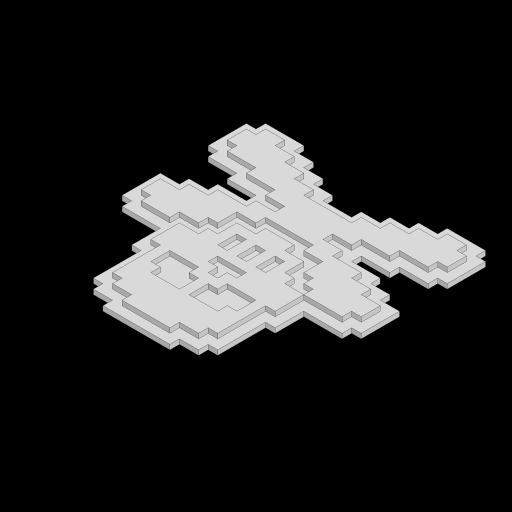
# Autodesk Inventor part: PKSkull
Saved by Autodesk Inventor 2023 (Build 270158000, 158)
## iProperties
Created: 2023-09-16
Part Number: PKSkull
Material: Generic
Document SubType Name: Modeling
Designer: tandu
Density: 1 g/cm^3
Appearance: Default
Author: tandu
Autodesk Inventor part; units mm, degrees
ref_plane "YZ Plane" through (0, 0, 0) normal (1, 0, 0) x (0, 1, 0)
ref_plane "XZ Plane" through (0, 0, 0) normal (0, 1, 0) x (-1, 0, 0)
ref_plane "XY Plane" through (0, 0, 0) normal (0, 0, 1) x (1, 0, 0)
sketch "Sketch1" plane through (0, 0, 0) normal (0, 1, 0) x (-1, 0, 0)
  line L0 (3708.4, 6832.6) -> (3708.4, 6705.6)
  line L1 (3708.4, 6705.6) -> (3454.4, 6705.6)
  line L2 (3454.4, 6705.6) -> (3200.4, 6705.6)
  line L3 (3200.4, 6705.6) -> (3200.4, 6578.6)
  line L4 (3200.4, 6578.6) -> (3200.4, 6451.6)
  line L5 (3200.4, 6451.6) -> (3073.4, 6451.6)
  line L6 (3073.4, 6451.6) -> (2946.4, 6451.6)
  line L7 (2946.4, 6451.6) -> (2946.4, 5816.6)
  line L8 (2946.4, 5816.6) -> (2946.4, 5181.6)
  line L9 (2946.4, 5181.6) -> (2819.4, 5181.6)
  line L10 (2819.4, 5181.6) -> (2692.4, 5181.6)
  line L11 (2692.4, 5181.6) -> (2692.4, 4800.6)
  line L12 (2692.4, 4800.6) -> (2692.4, 4419.6)
  line L13 (2692.4, 4419.6) -> (2184.4, 4419.6)
  line L14 (2184.4, 4419.6) -> (1676.4, 4419.6)
  line L15 (1676.4, 4419.6) -> (1676.4, 4292.6)
  line L16 (1676.4, 4292.6) -> (1676.4, 4165.6)
  line L17 (1676.4, 4165.6) -> (1549.4, 4165.6)
  line L18 (1549.4, 4165.6) -> (1422.4, 4165.6)
  line L19 (1422.4, 4165.6) -> (1422.4, 3657.6)
  line L20 (1422.4, 3657.6) -> (1422.4, 3149.6)
  line L21 (1422.4, 3149.6) -> (1676.4, 3149.6)
  line L22 (1676.4, 3149.6) -> (1930.4, 3149.6)
  line L23 (1930.4, 3149.6) -> (1930.4, 3022.6)
  line L24 (1930.4, 3022.6) -> (1930.4, 2895.6)
  line L25 (1930.4, 2895.6) -> (2184.4, 2895.6)
  line L26 (2184.4, 2895.6) -> (2438.4, 2895.6)
  line L27 (2438.4, 2895.6) -> (2438.4, 2768.6)
  line L28 (2438.4, 2768.6) -> (2438.4, 2641.6)
  line L29 (2438.4, 2641.6) -> (2819.4, 2641.6)
  line L30 (2819.4, 2641.6) -> (3200.4, 2641.6)
  line L31 (3200.4, 2641.6) -> (3200.4, 2514.6)
  line L32 (3200.4, 2514.6) -> (3200.4, 2387.6)
  line L33 (3200.4, 2387.6) -> (2819.4, 2387.6)
  line L34 (2819.4, 2387.6) -> (2438.4, 2387.6)
  line L35 (2438.4, 2387.6) -> (2438.4, 2260.6)
  line L36 (2438.4, 2260.6) -> (2438.4, 2133.6)
  line L37 (2438.4, 2133.6) -> (2057.4, 2133.6)
  line L38 (2057.4, 2133.6) -> (1676.4, 2133.6)
  line L39 (1676.4, 2133.6) -> (1676.4, 2006.6)
  line L40 (1676.4, 2006.6) -> (1676.4, 1879.6)
  line L41 (1676.4, 1879.6) -> (1549.4, 1879.6)
  line L42 (1549.4, 1879.6) -> (1422.4, 1879.6)
  line L43 (1422.4, 1879.6) -> (1422.4, 1371.6)
  line L44 (1422.4, 1371.6) -> (1422.4, 863.6)
  line L45 (1422.4, 863.6) -> (1549.4, 863.6)
  line L46 (1549.4, 863.6) -> (1676.4, 863.6)
  line L47 (1676.4, 863.6) -> (1676.4, 736.6)
  line L48 (1676.4, 736.6) -> (1676.4, 609.6)
  line L49 (1676.4, 609.6) -> (2184.4, 609.6)
  line L50 (2184.4, 609.6) -> (2692.4, 609.6)
  line L51 (2692.4, 609.6) -> (2692.4, 736.6)
  line L52 (2692.4, 736.6) -> (2692.4, 863.6)
  line L53 (2692.4, 863.6) -> (2946.4, 863.6)
  line L54 (2946.4, 863.6) -> (3200.4, 863.6)
  line L55 (3200.4, 863.6) -> (3200.4, 990.6)
  line L56 (3200.4, 990.6) -> (3200.4, 1117.6)
  line L57 (3200.4, 1117.6) -> (3454.4, 1117.6)
  line L58 (3454.4, 1117.6) -> (3708.4, 1117.6)
  line L59 (3708.4, 1117.6) -> (3708.4, 1244.6)
  line L60 (3708.4, 1244.6) -> (3708.4, 1371.6)
  line L61 (3708.4, 1371.6) -> (3962.4, 1371.6)
  line L62 (3962.4, 1371.6) -> (4216.4, 1371.6)
  line L63 (4216.4, 1371.6) -> (4216.4, 1498.6)
  line L64 (4216.4, 1498.6) -> (4216.4, 1625.6)
  line L65 (4216.4, 1625.6) -> (4597.4, 1625.6)
  line L66 (4597.4, 1625.6) -> (4978.4, 1625.6)
  line L67 (4978.4, 1625.6) -> (4978.4, 1498.6)
  line L68 (4978.4, 1498.6) -> (4978.4, 1371.6)
  line L69 (4978.4, 1371.6) -> (5232.4, 1371.6)
  line L70 (5232.4, 1371.6) -> (5486.4, 1371.6)
  line L71 (5486.4, 1371.6) -> (5486.4, 1244.6)
  line L72 (5486.4, 1244.6) -> (5486.4, 1117.6)
  line L73 (5486.4, 1117.6) -> (5740.4, 1117.6)
  line L74 (5740.4, 1117.6) -> (5994.4, 1117.6)
  line L75 (5994.4, 1117.6) -> (5994.4, 990.6)
  line L76 (5994.4, 990.6) -> (5994.4, 863.6)
  line L77 (5994.4, 863.6) -> (6248.4, 863.6)
  line L78 (6248.4, 863.6) -> (6502.4, 863.6)
  line L79 (6502.4, 863.6) -> (6502.4, 736.6)
  line L80 (6502.4, 736.6) -> (6502.4, 609.6)
  line L81 (6502.4, 609.6) -> (7010.4, 609.6)
  line L82 (7010.4, 609.6) -> (7518.4, 609.6)
  line L83 (7518.4, 609.6) -> (7518.4, 736.6)
  line L84 (7518.4, 736.6) -> (7518.4, 863.6)
  line L85 (7518.4, 863.6) -> (7645.4, 863.6)
  line L86 (7645.4, 863.6) -> (7772.4, 863.6)
  line L87 (7772.4, 863.6) -> (7772.4, 1371.6)
  line L88 (7772.4, 1371.6) -> (7772.4, 1879.6)
  line L89 (7772.4, 1879.6) -> (7645.4, 1879.6)
  line L90 (7645.4, 1879.6) -> (7518.4, 1879.6)
  line L91 (7518.4, 1879.6) -> (7518.4, 2006.6)
  line L92 (7518.4, 2006.6) -> (7518.4, 2133.6)
  line L93 (7518.4, 2133.6) -> (7137.4, 2133.6)
  line L94 (7137.4, 2133.6) -> (6756.4, 2133.6)
  line L95 (6756.4, 2133.6) -> (6756.4, 2260.6)
  line L96 (6756.4, 2260.6) -> (6756.4, 2387.6)
  line L97 (6756.4, 2387.6) -> (6375.4, 2387.6)
  line L98 (6375.4, 2387.6) -> (5994.4, 2387.6)
  line L99 (5994.4, 2387.6) -> (5994.4, 2514.6)
  line L100 (5994.4, 2514.6) -> (5994.4, 2641.6)
  line L101 (5994.4, 2641.6) -> (6375.4, 2641.6)
  line L102 (6375.4, 2641.6) -> (6756.4, 2641.6)
  line L103 (6756.4, 2641.6) -> (6756.4, 2768.6)
  line L104 (6756.4, 2768.6) -> (6756.4, 2895.6)
  line L105 (6756.4, 2895.6) -> (7010.4, 2895.6)
  line L106 (7010.4, 2895.6) -> (7264.4, 2895.6)
  line L107 (7264.4, 2895.6) -> (7264.4, 3022.6)
  line L108 (7264.4, 3022.6) -> (7264.4, 3149.6)
  line L109 (7264.4, 3149.6) -> (7518.4, 3149.6)
  line L110 (7518.4, 3149.6) -> (7772.4, 3149.6)
  line L111 (7772.4, 3149.6) -> (7772.4, 3657.6)
  line L112 (7772.4, 3657.6) -> (7772.4, 4165.6)
  line L113 (7772.4, 4165.6) -> (7645.4, 4165.6)
  line L114 (7645.4, 4165.6) -> (7518.4, 4165.6)
  line L115 (7518.4, 4165.6) -> (7518.4, 4292.6)
  line L116 (7518.4, 4292.6) -> (7518.4, 4419.6)
  line L117 (7518.4, 4419.6) -> (7010.4, 4419.6)
  line L118 (7010.4, 4419.6) -> (6502.4, 4419.6)
  line L119 (6502.4, 4419.6) -> (6502.4, 4800.6)
  line L120 (6502.4, 4800.6) -> (6502.4, 5181.6)
  line L121 (6502.4, 5181.6) -> (6375.4, 5181.6)
  line L122 (6375.4, 5181.6) -> (6248.4, 5181.6)
  line L123 (6248.4, 5181.6) -> (6248.4, 5816.6)
  line L124 (6248.4, 5816.6) -> (6248.4, 6451.6)
  line L125 (6248.4, 6451.6) -> (6121.4, 6451.6)
  line L126 (6121.4, 6451.6) -> (5994.4, 6451.6)
  line L127 (5994.4, 6451.6) -> (5994.4, 6578.6)
  line L128 (5994.4, 6578.6) -> (5994.4, 6705.6)
  line L129 (5994.4, 6705.6) -> (5740.4, 6705.6)
  line L130 (5740.4, 6705.6) -> (5486.4, 6705.6)
  line L131 (5486.4, 6705.6) -> (5486.4, 6832.6)
  line L132 (5486.4, 6832.6) -> (5486.4, 6959.6)
  line L133 (5486.4, 6959.6) -> (4597.4, 6959.6)
  line L134 (4597.4, 6959.6) -> (3708.4, 6959.6)
  line L135 (3708.4, 6959.6) -> (3708.4, 6832.6)
  line L136 (5232.4, 6578.6) -> (5232.4, 6451.6)
  line L137 (5232.4, 6451.6) -> (5486.4, 6451.6)
  line L138 (5486.4, 6451.6) -> (5740.4, 6451.6)
  line L139 (5740.4, 6451.6) -> (5740.4, 6324.6)
  line L140 (5740.4, 6324.6) -> (5740.4, 6197.6)
  line L141 (5740.4, 6197.6) -> (5867.4, 6197.6)
  line L142 (5867.4, 6197.6) -> (5994.4, 6197.6)
  line L143 (5994.4, 6197.6) -> (5994.4, 5562.6)
  line L144 (5994.4, 5562.6) -> (5994.4, 4927.6)
  line L145 (5994.4, 4927.6) -> (6121.4, 4927.6)
  line L146 (6121.4, 4927.6) -> (6248.4, 4927.6)
  line L147 (6248.4, 4927.6) -> (6248.4, 4546.6)
  line L148 (6248.4, 4546.6) -> (6248.4, 4165.6)
  line L149 (6248.4, 4165.6) -> (5994.4, 4165.6)
  line L150 (5994.4, 4165.6) -> (5740.4, 4165.6)
  line L151 (5740.4, 4165.6) -> (5740.4, 4038.6)
  line L152 (5740.4, 4038.6) -> (5740.4, 3911.6)
  line L153 (5740.4, 3911.6) -> (5613.4, 3911.6)
  line L154 (5613.4, 3911.6) -> (5486.4, 3911.6)
  line L155 (5486.4, 3911.6) -> (5486.4, 3657.6)
  line L156 (5486.4, 3657.6) -> (5486.4, 3403.6)
  line L157 (5486.4, 3403.6) -> (5232.4, 3403.6)
  line L158 (5232.4, 3403.6) -> (4978.4, 3403.6)
  line L159 (4978.4, 3403.6) -> (4978.4, 3276.6)
  line L160 (4978.4, 3276.6) -> (4978.4, 3149.6)
  line L161 (4978.4, 3149.6) -> (4597.4, 3149.6)
  line L162 (4597.4, 3149.6) -> (4216.4, 3149.6)
  line L163 (4216.4, 3149.6) -> (4216.4, 3276.6)
  line L164 (4216.4, 3276.6) -> (4216.4, 3403.6)
  line L165 (4216.4, 3403.6) -> (3962.4, 3403.6)
  line L166 (3962.4, 3403.6) -> (3708.4, 3403.6)
  line L167 (3708.4, 3403.6) -> (3708.4, 3657.6)
  line L168 (3708.4, 3657.6) -> (3708.4, 3911.6)
  line L169 (3708.4, 3911.6) -> (3581.4, 3911.6)
  line L170 (3581.4, 3911.6) -> (3454.4, 3911.6)
  line L171 (3454.4, 3911.6) -> (3454.4, 4038.6)
  line L172 (3454.4, 4038.6) -> (3454.4, 4165.6)
  line L173 (3454.4, 4165.6) -> (3200.4, 4165.6)
  line L174 (3200.4, 4165.6) -> (2946.4, 4165.6)
  line L175 (2946.4, 4165.6) -> (2946.4, 4038.6)
  line L176 (2946.4, 4038.6) -> (2946.4, 3911.6)
  line L177 (2946.4, 3911.6) -> (3073.4, 3911.6)
  line L178 (3073.4, 3911.6) -> (3200.4, 3911.6)
  line L179 (3200.4, 3911.6) -> (3200.4, 3784.6)
  line L180 (3200.4, 3784.6) -> (3200.4, 3657.6)
  line L181 (3200.4, 3657.6) -> (3327.4, 3657.6)
  line L182 (3327.4, 3657.6) -> (3454.4, 3657.6)
  line L183 (3454.4, 3657.6) -> (3454.4, 3403.6)
  line L184 (3454.4, 3403.6) -> (3454.4, 3149.6)
  line L185 (3454.4, 3149.6) -> (3708.4, 3149.6)
  line L186 (3708.4, 3149.6) -> (3962.4, 3149.6)
  line L187 (3962.4, 3149.6) -> (3962.4, 3022.6)
  line L188 (3962.4, 3022.6) -> (3962.4, 2895.6)
  line L189 (3962.4, 2895.6) -> (4597.4, 2895.6)
  line L190 (4597.4, 2895.6) -> (5232.4, 2895.6)
  line L191 (5232.4, 2895.6) -> (5232.4, 3022.6)
  line L192 (5232.4, 3022.6) -> (5232.4, 3149.6)
  line L193 (5232.4, 3149.6) -> (5486.4, 3149.6)
  line L194 (5486.4, 3149.6) -> (5740.4, 3149.6)
  line L195 (5740.4, 3149.6) -> (5740.4, 3403.6)
  line L196 (5740.4, 3403.6) -> (5740.4, 3657.6)
  line L197 (5740.4, 3657.6) -> (5867.4, 3657.6)
  line L198 (5867.4, 3657.6) -> (5994.4, 3657.6)
  line L199 (5994.4, 3657.6) -> (5994.4, 3784.6)
  line L200 (5994.4, 3784.6) -> (5994.4, 3911.6)
  line L201 (5994.4, 3911.6) -> (6248.4, 3911.6)
  line L202 (6248.4, 3911.6) -> (6502.4, 3911.6)
  line L203 (6502.4, 3911.6) -> (6502.4, 4038.6)
  line L204 (6502.4, 4038.6) -> (6502.4, 4165.6)
  line L205 (6502.4, 4165.6) -> (6883.4, 4165.6)
  line L206 (6883.4, 4165.6) -> (7264.4, 4165.6)
  line L207 (7264.4, 4165.6) -> (7264.4, 4038.6)
  line L208 (7264.4, 4038.6) -> (7264.4, 3911.6)
  line L209 (7264.4, 3911.6) -> (7391.4, 3911.6)
  line L210 (7391.4, 3911.6) -> (7518.4, 3911.6)
  line L211 (7518.4, 3911.6) -> (7518.4, 3657.6)
  line L212 (7518.4, 3657.6) -> (7518.4, 3403.6)
  line L213 (7518.4, 3403.6) -> (7264.4, 3403.6)
  line L214 (7264.4, 3403.6) -> (7010.4, 3403.6)
  line L215 (7010.4, 3403.6) -> (7010.4, 3276.6)
  line L216 (7010.4, 3276.6) -> (7010.4, 3149.6)
  line L217 (7010.4, 3149.6) -> (6756.4, 3149.6)
  line L218 (6756.4, 3149.6) -> (6502.4, 3149.6)
  line L219 (6502.4, 3149.6) -> (6502.4, 3022.6)
  line L220 (6502.4, 3022.6) -> (6502.4, 2895.6)
  line L221 (6502.4, 2895.6) -> (6121.4, 2895.6)
  line L222 (6121.4, 2895.6) -> (5740.4, 2895.6)
  line L223 (5740.4, 2895.6) -> (5740.4, 2768.6)
  line L224 (5740.4, 2768.6) -> (5740.4, 2641.6)
  line L225 (5740.4, 2641.6) -> (5486.4, 2641.6)
  line L226 (5486.4, 2641.6) -> (5232.4, 2641.6)
  line L227 (5232.4, 2641.6) -> (5232.4, 2514.6)
  line L228 (5232.4, 2514.6) -> (5232.4, 2387.6)
  line L229 (5232.4, 2387.6) -> (5486.4, 2387.6)
  line L230 (5486.4, 2387.6) -> (5740.4, 2387.6)
  line L231 (5740.4, 2387.6) -> (5740.4, 2260.6)
  line L232 (5740.4, 2260.6) -> (5740.4, 2133.6)
  line L233 (5740.4, 2133.6) -> (6121.4, 2133.6)
  line L234 (6121.4, 2133.6) -> (6502.4, 2133.6)
  line L235 (6502.4, 2133.6) -> (6502.4, 2006.6)
  line L236 (6502.4, 2006.6) -> (6502.4, 1879.6)
  line L237 (6502.4, 1879.6) -> (6883.4, 1879.6)
  line L238 (6883.4, 1879.6) -> (7264.4, 1879.6)
  line L239 (7264.4, 1879.6) -> (7264.4, 1752.6)
  line L240 (7264.4, 1752.6) -> (7264.4, 1625.6)
  line L241 (7264.4, 1625.6) -> (7391.4, 1625.6)
  line L242 (7391.4, 1625.6) -> (7518.4, 1625.6)
  line L243 (7518.4, 1625.6) -> (7518.4, 1371.6)
  line L244 (7518.4, 1371.6) -> (7518.4, 1117.6)
  line L245 (7518.4, 1117.6) -> (7391.4, 1117.6)
  line L246 (7391.4, 1117.6) -> (7264.4, 1117.6)
  line L247 (7264.4, 1117.6) -> (7264.4, 990.6)
  line L248 (7264.4, 990.6) -> (7264.4, 863.6)
  line L249 (7264.4, 863.6) -> (7010.4, 863.6)
  line L250 (7010.4, 863.6) -> (6756.4, 863.6)
  line L251 (6756.4, 863.6) -> (6756.4, 990.6)
  line L252 (6756.4, 990.6) -> (6756.4, 1117.6)
  line L253 (6756.4, 1117.6) -> (6502.4, 1117.6)
  line L254 (6502.4, 1117.6) -> (6248.4, 1117.6)
  line L255 (6248.4, 1117.6) -> (6248.4, 1244.6)
  line L256 (6248.4, 1244.6) -> (6248.4, 1371.6)
  line L257 (6248.4, 1371.6) -> (5994.4, 1371.6)
  line L258 (5994.4, 1371.6) -> (5740.4, 1371.6)
  line L259 (5740.4, 1371.6) -> (5740.4, 1498.6)
  line L260 (5740.4, 1498.6) -> (5740.4, 1625.6)
  line L261 (5740.4, 1625.6) -> (5486.4, 1625.6)
  line L262 (5486.4, 1625.6) -> (5232.4, 1625.6)
  line L263 (5232.4, 1625.6) -> (5232.4, 1752.6)
  line L264 (5232.4, 1752.6) -> (5232.4, 1879.6)
  line L265 (5232.4, 1879.6) -> (4597.4, 1879.6)
  line L266 (4597.4, 1879.6) -> (3962.4, 1879.6)
  line L267 (3962.4, 1879.6) -> (3962.4, 1752.6)
  line L268 (3962.4, 1752.6) -> (3962.4, 1625.6)
  line L269 (3962.4, 1625.6) -> (3708.4, 1625.6)
  line L270 (3708.4, 1625.6) -> (3454.4, 1625.6)
  line L271 (3454.4, 1625.6) -> (3454.4, 1498.6)
  line L272 (3454.4, 1498.6) -> (3454.4, 1371.6)
  line L273 (3454.4, 1371.6) -> (3200.4, 1371.6)
  line L274 (3200.4, 1371.6) -> (2946.4, 1371.6)
  line L275 (2946.4, 1371.6) -> (2946.4, 1244.6)
  line L276 (2946.4, 1244.6) -> (2946.4, 1117.6)
  line L277 (2946.4, 1117.6) -> (2692.4, 1117.6)
  line L278 (2692.4, 1117.6) -> (2438.4, 1117.6)
  line L279 (2438.4, 1117.6) -> (2438.4, 990.6)
  line L280 (2438.4, 990.6) -> (2438.4, 863.6)
  line L281 (2438.4, 863.6) -> (2184.4, 863.6)
  line L282 (2184.4, 863.6) -> (1930.4, 863.6)
  line L283 (1930.4, 863.6) -> (1930.4, 990.6)
  line L284 (1930.4, 990.6) -> (1930.4, 1117.6)
  line L285 (1930.4, 1117.6) -> (1803.4, 1117.6)
  line L286 (1803.4, 1117.6) -> (1676.4, 1117.6)
  line L287 (1676.4, 1117.6) -> (1676.4, 1371.6)
  line L288 (1676.4, 1371.6) -> (1676.4, 1625.6)
  line L289 (1676.4, 1625.6) -> (1803.4, 1625.6)
  line L290 (1803.4, 1625.6) -> (1930.4, 1625.6)
  line L291 (1930.4, 1625.6) -> (1930.4, 1752.6)
  line L292 (1930.4, 1752.6) -> (1930.4, 1879.6)
  line L293 (1930.4, 1879.6) -> (2311.4, 1879.6)
  line L294 (2311.4, 1879.6) -> (2692.4, 1879.6)
  line L295 (2692.4, 1879.6) -> (2692.4, 2006.6)
  line L296 (2692.4, 2006.6) -> (2692.4, 2133.6)
  line L297 (2692.4, 2133.6) -> (3073.4, 2133.6)
  line L298 (3073.4, 2133.6) -> (3454.4, 2133.6)
  line L299 (3454.4, 2133.6) -> (3454.4, 2260.6)
  line L300 (3454.4, 2260.6) -> (3454.4, 2387.6)
  line L301 (3454.4, 2387.6) -> (3708.4, 2387.6)
  line L302 (3708.4, 2387.6) -> (3962.4, 2387.6)
  line L303 (3962.4, 2387.6) -> (3962.4, 2514.6)
  line L304 (3962.4, 2514.6) -> (3962.4, 2641.6)
  line L305 (3962.4, 2641.6) -> (3708.4, 2641.6)
  line L306 (3708.4, 2641.6) -> (3454.4, 2641.6)
  line L307 (3454.4, 2641.6) -> (3454.4, 2768.6)
  line L308 (3454.4, 2768.6) -> (3454.4, 2895.6)
  line L309 (3454.4, 2895.6) -> (3073.4, 2895.6)
  line L310 (3073.4, 2895.6) -> (2692.4, 2895.6)
  line L311 (2692.4, 2895.6) -> (2692.4, 3022.6)
  line L312 (2692.4, 3022.6) -> (2692.4, 3149.6)
  line L313 (2692.4, 3149.6) -> (2438.4, 3149.6)
  line L314 (2438.4, 3149.6) -> (2184.4, 3149.6)
  line L315 (2184.4, 3149.6) -> (2184.4, 3276.6)
  line L316 (2184.4, 3276.6) -> (2184.4, 3403.6)
  line L317 (2184.4, 3403.6) -> (1930.4, 3403.6)
  line L318 (1930.4, 3403.6) -> (1676.4, 3403.6)
  line L319 (1676.4, 3403.6) -> (1676.4, 3657.6)
  line L320 (1676.4, 3657.6) -> (1676.4, 3911.6)
  line L321 (1676.4, 3911.6) -> (1803.4, 3911.6)
  line L322 (1803.4, 3911.6) -> (1930.4, 3911.6)
  line L323 (1930.4, 3911.6) -> (1930.4, 4038.6)
  line L324 (1930.4, 4038.6) -> (1930.4, 4165.6)
  line L325 (1930.4, 4165.6) -> (2438.4, 4165.6)
  line L326 (2438.4, 4165.6) -> (2946.4, 4165.6)
  line L327 (2946.4, 4165.6) -> (2946.4, 4546.6)
  line L328 (2946.4, 4546.6) -> (2946.4, 4927.6)
  line L329 (2946.4, 4927.6) -> (3073.4, 4927.6)
  line L330 (3073.4, 4927.6) -> (3200.4, 4927.6)
  line L331 (3200.4, 4927.6) -> (3200.4, 5562.6)
  line L332 (3200.4, 5562.6) -> (3200.4, 6197.6)
  line L333 (3200.4, 6197.6) -> (3327.4, 6197.6)
  line L334 (3327.4, 6197.6) -> (3454.4, 6197.6)
  line L335 (3454.4, 6197.6) -> (3454.4, 6324.6)
  line L336 (3454.4, 6324.6) -> (3454.4, 6451.6)
  line L337 (3454.4, 6451.6) -> (3708.4, 6451.6)
  line L338 (3708.4, 6451.6) -> (3962.4, 6451.6)
  line L339 (3962.4, 6451.6) -> (3962.4, 6578.6)
  line L340 (3962.4, 6578.6) -> (3962.4, 6705.6)
  line L341 (3962.4, 6705.6) -> (4597.4, 6705.6)
  line L342 (4597.4, 6705.6) -> (5232.4, 6705.6)
  line L343 (5232.4, 6705.6) -> (5232.4, 6578.6)
  line L344 (3708.4, 5562.6) -> (3708.4, 5435.6)
  line L345 (3708.4, 5435.6) -> (3581.4, 5435.6)
  line L346 (3581.4, 5435.6) -> (3454.4, 5435.6)
  line L347 (3454.4, 5435.6) -> (3454.4, 5181.6)
  line L348 (3454.4, 5181.6) -> (3454.4, 4927.6)
  line L349 (3454.4, 4927.6) -> (3835.4, 4927.6)
  line L350 (3835.4, 4927.6) -> (4216.4, 4927.6)
  line L351 (4216.4, 4927.6) -> (4216.4, 5054.6)
  line L352 (4216.4, 5054.6) -> (4216.4, 5181.6)
  line L353 (4216.4, 5181.6) -> (4343.4, 5181.6)
  line L354 (4343.4, 5181.6) -> (4470.4, 5181.6)
  line L355 (4470.4, 5181.6) -> (4470.4, 5435.6)
  line L356 (4470.4, 5435.6) -> (4470.4, 5689.6)
  line L357 (4470.4, 5689.6) -> (4089.4, 5689.6)
  line L358 (4089.4, 5689.6) -> (3708.4, 5689.6)
  line L359 (3708.4, 5689.6) -> (3708.4, 5562.6)
  line L360 (4724.4, 5435.6) -> (4724.4, 5181.6)
  line L361 (4724.4, 5181.6) -> (4851.4, 5181.6)
  line L362 (4851.4, 5181.6) -> (4978.4, 5181.6)
  line L363 (4978.4, 5181.6) -> (4978.4, 5054.6)
  line L364 (4978.4, 5054.6) -> (4978.4, 4927.6)
  line L365 (4978.4, 4927.6) -> (5359.4, 4927.6)
  line L366 (5359.4, 4927.6) -> (5740.4, 4927.6)
  line L367 (5740.4, 4927.6) -> (5740.4, 5181.6)
  line L368 (5740.4, 5181.6) -> (5740.4, 5435.6)
  line L369 (5740.4, 5435.6) -> (5613.4, 5435.6)
  line L370 (5613.4, 5435.6) -> (5486.4, 5435.6)
  line L371 (5486.4, 5435.6) -> (5486.4, 5562.6)
  line L372 (5486.4, 5562.6) -> (5486.4, 5689.6)
  line L373 (5486.4, 5689.6) -> (5105.4, 5689.6)
  line L374 (5105.4, 5689.6) -> (4724.4, 5689.6)
  line L375 (4724.4, 5689.6) -> (4724.4, 5435.6)
  line L376 (4470.4, 4800.6) -> (4470.4, 4673.6)
  line L377 (4470.4, 4673.6) -> (4343.4, 4673.6)
  line L378 (4343.4, 4673.6) -> (4216.4, 4673.6)
  line L379 (4216.4, 4673.6) -> (4216.4, 4546.6)
  line L380 (4216.4, 4546.6) -> (4216.4, 4419.6)
  line L381 (4216.4, 4419.6) -> (4597.4, 4419.6)
  line L382 (4597.4, 4419.6) -> (4978.4, 4419.6)
  line L383 (4978.4, 4419.6) -> (4978.4, 4546.6)
  line L384 (4978.4, 4546.6) -> (4978.4, 4673.6)
  line L385 (4978.4, 4673.6) -> (4851.4, 4673.6)
  line L386 (4851.4, 4673.6) -> (4724.4, 4673.6)
  line L387 (4724.4, 4673.6) -> (4724.4, 4800.6)
  line L388 (4724.4, 4800.6) -> (4724.4, 4927.6)
  line L389 (4724.4, 4927.6) -> (4597.4, 4927.6)
  line L390 (4597.4, 4927.6) -> (4470.4, 4927.6)
  line L391 (4470.4, 4927.6) -> (4470.4, 4800.6)
  line L392 (3962.4, 3911.6) -> (3962.4, 3657.6)
  line L393 (3962.4, 3657.6) -> (4089.4, 3657.6)
  line L394 (4089.4, 3657.6) -> (4216.4, 3657.6)
  line L395 (4216.4, 3657.6) -> (4216.4, 3911.6)
  line L396 (4216.4, 3911.6) -> (4216.4, 4165.6)
  line L397 (4216.4, 4165.6) -> (4089.4, 4165.6)
  line L398 (4089.4, 4165.6) -> (3962.4, 4165.6)
  line L399 (3962.4, 4165.6) -> (3962.4, 3911.6)
  line L400 (4470.4, 3911.6) -> (4470.4, 3657.6)
  line L401 (4470.4, 3657.6) -> (4597.4, 3657.6)
  line L402 (4597.4, 3657.6) -> (4724.4, 3657.6)
  line L403 (4724.4, 3657.6) -> (4724.4, 3911.6)
  line L404 (4724.4, 3911.6) -> (4724.4, 4165.6)
  line L405 (4724.4, 4165.6) -> (4597.4, 4165.6)
  line L406 (4597.4, 4165.6) -> (4470.4, 4165.6)
  line L407 (4470.4, 4165.6) -> (4470.4, 3911.6)
  line L408 (4978.4, 3911.6) -> (4978.4, 3657.6)
  line L409 (4978.4, 3657.6) -> (5105.4, 3657.6)
  line L410 (5105.4, 3657.6) -> (5232.4, 3657.6)
  line L411 (5232.4, 3657.6) -> (5232.4, 3911.6)
  line L412 (5232.4, 3911.6) -> (5232.4, 4165.6)
  line L413 (5232.4, 4165.6) -> (5105.4, 4165.6)
  line L414 (5105.4, 4165.6) -> (4978.4, 4165.6)
  line L415 (4978.4, 4165.6) -> (4978.4, 3911.6)
  point P0 (0, 0)
  constraints: 832 end point
extrude "Base" add sketch "Sketch1" against normal blind 127 contours L135 L134 L133 L132 L131 L130 L129 L128 L127 L126 L125 L124 L123 L122 L121 L120 L119 L118 L117 L116 L115 L114 L113 L112 L111 L110 L109 L108 L107 L106 L105 L104 L103 L102 L101 L100 L99 L98 L97 L96 L95 L94 L93 L92 L91 L90 L89 L88 L87 L86 L85 L84 L83 L82 L81 L80 L79 L78 L77 L76 L75 L74 L73 L72 L71 L70 L69 L68 L67 L66 L65 L64 L63 L62 L61 L60 L59 L58 L57 L56 L55 L54 L53 L52 L51 L50 L49 L48 L47 L46 L45 L44 L43 L42 L41 L40 L39 L38 L37 L36 L35 L34 L33 L32 L31 L30 L29 L28 L27 L26 L25 L24 L23 L22 L21 L20 L19 L18 L17 L16 L15 L14 L13 L12 L11 L10 L9 L8 L7 L6 L5 L4 L3 L2 L1 L0 | L175 L176 L177 L178 L179 L180 L181 L182 L183 L184 L185 L186 L187 L188 L189 L190 L191 L192 L193 L194 L195 L196 L197 L198 L199 L200 L201 L202 L203 L204 L205 L206 L207 L208 L209 L210 L211 L212 L213 L214 L215 L216 L217 L218 L219 L220 L221 L222 L223 L224 L225 L226 L227 L228 L229 L230 L231 L232 L233 L234 L235 L236 L237 L238 L239 L240 L241 L242 L243 L244 L245 L246 L247 L248 L249 L250 L251 L252 L253 L254 L255 L256 L257 L258 L259 L260 L261 L262 L263 L264 L265 L266 L267 L268 L269 L270 L271 L272 L273 L274 L275 L276 L277 L278 L279 L280 L281 L282 L283 L284 L285 L286 L287 L288 L289 L290 L291 L292 L293 L294 L295 L296 L297 L298 L299 L300 L301 L302 L303 L304 L305 L306 L307 L308 L309 L310 L311 L312 L313 L314 L315 L316 L317 L318 L319 L320 L321 L322 L323 L324 L325 L326 | L136 L137 L138 L139 L140 L141 L142 L143 L144 L145 L146 L147 L148 L149 L150 L151 L152 L153 L154 L155 L156 L157 L158 L159 L160 L161 L162 L163 L164 L165 L166 L167 L168 L169 L170 L171 L172 L173 L174 L327 L328 L329 L330 L331 L332 L333 L334 L335 L336 L337 L338 L339 L340 L341 L342 L343 | L359 L358 L357 L356 L355 L354 L353 L352 L351 L350 L349 L348 L347 L346 L345 L344 | L375 L374 L373 L372 L371 L370 L369 L368 L367 L366 L365 L364 L363 L362 L361 L360 | L391 L390 L389 L388 L387 L386 L385 L384 L383 L382 L381 L380 L379 L378 L377 L376 | L399 L398 L397 L396 L395 L394 L393 L392 | L407 L406 L405 L404 L403 L402 L401 L400 | L415 L414 L413 L412 L411 L410 L409 L408
extrude "Extrusion2" add sketch "Sketch1" along normal blind 127 contours L175 L176 L177 L178 L179 L180 L181 L182 L183 L184 L185 L186 L187 L188 L189 L190 L191 L192 L193 L194 L195 L196 L197 L198 L199 L200 L201 L202 L203 L204 L205 L206 L207 L208 L209 L210 L211 L212 L213 L214 L215 L216 L217 L218 L219 L220 L221 L222 L223 L224 L225 L226 L227 L228 L229 L230 L231 L232 L233 L234 L235 L236 L237 L238 L239 L240 L241 L242 L243 L244 L245 L246 L247 L248 L249 L250 L251 L252 L253 L254 L255 L256 L257 L258 L259 L260 L261 L262 L263 L264 L265 L266 L267 L268 L269 L270 L271 L272 L273 L274 L275 L276 L277 L278 L279 L280 L281 L282 L283 L284 L285 L286 L287 L288 L289 L290 L291 L292 L293 L294 L295 L296 L297 L298 L299 L300 L301 L302 L303 L304 L305 L306 L307 L308 L309 L310 L311 L312 L313 L314 L315 L316 L317 L318 L319 L320 L321 L322 L323 L324 L325 L326 | L136 L137 L138 L139 L140 L141 L142 L143 L144 L145 L146 L147 L148 L149 L150 L151 L152 L153 L154 L155 L156 L157 L158 L159 L160 L161 L162 L163 L164 L165 L166 L167 L168 L169 L170 L171 L172 L173 L174 L327 L328 L329 L330 L331 L332 L333 L334 L335 L336 L337 L338 L339 L340 L341 L342 L343
body "Solid1"
